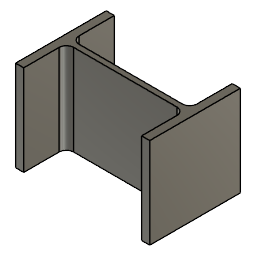
H-148×100×6×9 (Autodesk Fusion 360 design; units mm, degrees)
Autodesk Fusion 360 part; units mm, degrees
sketch "スケッチ1" plane through (0, 0, 0) normal (0, 0, 1) x (1, 0, 0)
  line L0 (0, 50) -> (0, -50)
  line L1 (148, -50) -> (148, 50)
  line L2 (17, -3) -> (131, -3)
  line L3 (9, -50) -> (9, -11)
  line L4 (0, -50) -> (9, -50)
  line L5 (139, -11) -> (139, -50)
  line L6 (139, -50) -> (148, -50)
  line L7 (131, 3) -> (17, 3)
  line L8 (9, 11) -> (9, 50)
  line L9 (9, 50) -> (0, 50)
  line L10 (139, 50) -> (139, 11)
  line L11 (148, 50) -> (139, 50)
  arc A0 (9, 11) -> (17, 3) centre (17, 11) ccw
  arc A1 (17, -3) -> (9, -11) centre (17, -11) ccw
  arc A2 (139, -11) -> (131, -3) centre (131, -11) ccw
  arc A3 (131, 3) -> (139, 11) centre (131, 11) ccw
extrude "押し出し1" add sketch "スケッチ1" along normal blind 100
